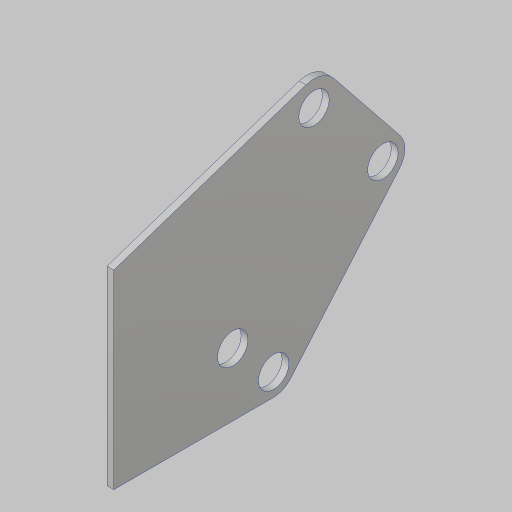
# Autodesk Inventor part: GI2 -001
Saved by Autodesk Inventor 2023.5 (Build 275446000, 446)
## iProperties
Created: 2025-01-25
Part Number: GI2 -001
Material: Aluminum 6061
Document SubType Name: Modeling
Designer: slick
Density: 2.7 g/cm^3
Appearance: Aluminum - Flat
Author: slick
Autodesk Inventor part; units mm, degrees
ref_plane "YZ Plane" through (0, 0, 0) normal (1, 0, 0) x (0, 1, 0)
ref_plane "XZ Plane" through (0, 0, 0) normal (0, 1, 0) x (-1, 0, 0)
ref_plane "XY Plane" through (0, 0, 0) normal (0, 0, 1) x (1, 0, 0)
sketch "Sketch1" plane through (0, 0, 0) normal (1, 0, 0) x (0, 1, 0)
  line L0 (0, 0) -> (50.8, 0) construction
  line L1 (50.8, 0) -> (50.8, 406.4) construction
  line L2 (50.8, 406.4) -> (0, 406.4) construction
  line L3 (0, 406.4) -> (0, 0) construction
  line L4 (-19.05, 406.4) -> (-19.05, 0) construction
  line L5 (127, 0) -> (-19.05, 0) construction
  line L6 (-19.05, 0) -> (-19.05, -76.2) construction
  line L7 (-19.05, -76.2) -> (127, -76.2) construction
  line L8 (127, -76.2) -> (127, 0) construction
  line L9 (7.9375, 127) -> (42.8625, 127) construction
  arc A0 (88.9, -76.2) -> (127, -38.1) centre (88.9, -38.1) ccw construction
  point P0 (25.4, 114.3)
  point P1 (25.4, 127)
  point P2 (25.4, 0)
  dimension "d0" = 50.8
  dimension "d1" = 406.4
  dimension "d2" = 19.05
  dimension "d3" = 146.05
  dimension "d4" = 76.2
  dimension "d5" = 34.925
  dimension "d6" = 114.3
  dimension "d7" = 12.7
  constraints: 20 end point, 5 parallel, 3 horizontal, 3 horizontal alignment, 3 midpoint, 2 perpendicular, 2 point on circle, 2 tangent, 2 vertical alignment, 1 centre point, 1 point on line, 1 vertical
  measures "d0" distance of L2.end L1.end
  measures "d1" distance of L1.end L0.end
  measures "d2" distance between parallel lines of L3 L4
  measures "d3" distance of L7.end L6.end
  measures "d4" distance of L4.end L6.end
  measures "d5" distance of L9.start L9.end
  measures "d6" distance from line of L0 point (25.4, 114.3)
  measures "d7" distance from line of point (25.4, 114.3) L9
sketch "Sketch2" plane through (0, 0, 0) normal (1, 0, 0) x (0, 1, 0)
  line L0 (0, 0) -> (50.8, 0) construction
  line L1 (50.8, 0) -> (50.8, 406.4) construction
  line L2 (50.8, 406.4) -> (0, 406.4) construction
  line L3 (0, 406.4) -> (0, 0) construction
  line L4 (-19.05, 406.4) -> (-19.05, 0) construction
  line L5 (-19.05, 0) -> (-19.05, -76.2) construction
  line L6 (7.9375, 127) -> (42.8625, 127) construction
  line L7 (127, 0) -> (-19.05, 0) construction
  line L8 (-19.05, -76.2) -> (127, -76.2) construction
  line L9 (127, -76.2) -> (127, 0) construction
  circle A0 centre (6.35, -149.3929) radius 17.4625 construction
  circle A1 centre (44.45, -111.125) radius 25.4 construction
  circle A2 centre (158.75, 86.4632) radius 57.15 construction
  circle A3 centre (125.73, -251.46) radius 38.1 construction
  circle A4 centre (38.2016, -220.3603) radius 57.15 construction
  circle A5 centre (44.45, -111.125) radius 19.05 construction
  circle A6 centre (200.9726, -187.1065) radius 38.1 construction
  circle A7 centre (200.9726, -187.1065) radius 31.75 construction
  circle A8 centre (125.73, -251.46) radius 31.75 construction
  circle A9 centre (78.1338, -179.4759) radius 57.15 construction
  arc A10 (88.9, -76.2) -> (127, -38.1) centre (88.9, -38.1) ccw construction
  circle A11 centre (200.9726, -187.1065) radius 14.2875
  circle A12 centre (125.73, -251.46) radius 14.2875
  circle A13 centre (6.35, -149.3929) radius 14.2875
  circle A14 centre (44.45, -111.125) radius 14.2875
  circle A15 centre (200.9726, -187.1065) radius 23.8125 construction
  circle A16 centre (125.73, -251.46) radius 20.6375 construction
  circle A17 centre (6.35, -149.3929) radius 20.6375 construction
  line L10 (215.8619, -205.69) -> (138.634, -267.5657)
  line L11 (112.3189, -267.1459) -> (-7.0611, -165.0789)
  line L12 (-14.2875, -149.3929) -> (-14.2875, 0)
  line L13 (-14.2875, 0) -> (163.5125, 0)
  line L14 (163.5125, 0) -> (223.5559, -179.5546)
  arc A18 (112.3189, -267.1459) -> (138.634, -267.5657) centre (125.73, -251.46) ccw
  arc A19 (-14.2875, -149.3929) -> (-7.0611, -165.0789) centre (6.35, -149.3929) ccw
  arc A20 (215.8619, -205.69) -> (223.5559, -179.5546) centre (200.9726, -187.1065) ccw
  point P0 (25.4, 127)
  point P1 (25.4, 0)
  point P2 (25.4, 114.3)
  dimension "d16" = 114.3
  dimension "d8" = 34.925
  dimension "d9" = 25.4
  dimension "d10" = 50.8
  dimension "d11" = 34.925
  dimension "d12" = 54.0004
  dimension "d13" = 63.5
  dimension "d14" = 114.3
  dimension "d15" = 76.2
  dimension "d17" = 6.35
  dimension "d18" = 76.2
  dimension "d19" = 6.35
  dimension "d20" = 6.35
  dimension "d21" = 114.3
  dimension "d22" = 99.0092
  dimension "d23" = 144.78
  dimension "d24" = 28.575
  dimension "d27" = 9.525
  dimension "d28" = 6.35
  dimension "d29" = 6.35
  dimension "d33" = 175.26
  dimension "d34" = 173.99
  dimension "d35" = 177.8
  constraints: 19 centre point, 12 point on circle, 10 end point, 7 coincident, 7 tangent, 4 equal radius, 1 collinear, 1 horizontal alignment, 1 point on line, 1 vertical, 4 other
  measures "d8" diameter of A0
  measures "d9" distance from line of A0.centre L5
  measures "d10" diameter of A1
  measures "d11" distance from line of A1.centre L8
  measures "d12" distance of A0.centre A1.centre
  measures "d13" distance from line of L5 A1.centre
  measures "d14" diameter of A2
  measures "d15" diameter of A3
  measures "d17" radial gap between concentric circles of A1 A5
  measures "d18" diameter of A6
  measures "d19" radial gap between concentric circles of A6 A7
  measures "d20" radial gap between concentric circles of A3 A8
  measures "d21" diameter of A9
  measures "d22" distance of A3.centre A6.centre
  measures "d23" distance from line of L5 A3.centre
  measures "d24" diameter of A11
  measures "d27" radial gap between concentric circles of A11 A15
  measures "d28" radial gap between concentric circles of A12 A16
  measures "d29" radial gap between concentric circles of A13 A17
  measures "d33" distance from line of A3.centre L8
  measures "d34" distance of A6.centre A1.centre
  measures "d35" distance of L12.end L13.end
extrude "Extrusion1" add sketch "Sketch2" along normal blind 6.35
body "Solid1"
